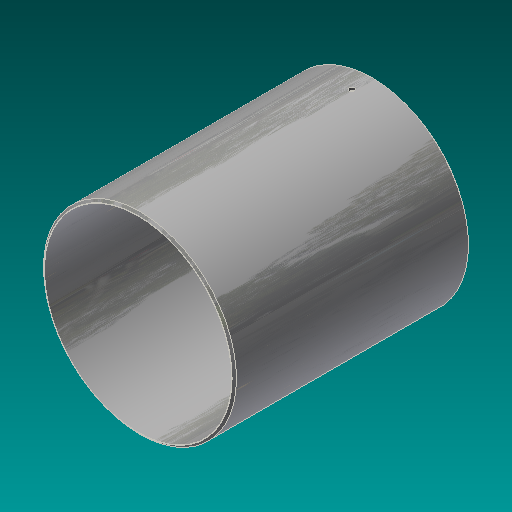
# Autodesk Inventor part: A1-19027-200-01 34in pipe
Saved by Autodesk Inventor 2017.3 (Build 213257000, 257)
## iProperties
Created: 2019-06-26
Part Number: A1-19027-200-01 34in pipe
Material: Steel, Mild
Document SubType Name: Modeling
Designer: Graeme_Van_Dongen
Density: 7.85 g/cm^3
Appearance: Steel
Mass: 279198 g
Surface Area: 56801.7 cm^2
Volume: 35566.7 cm^3
Description: 34" XS x 41 9/16" PIPE, API 5L X65M
Author: Graeme_Van_Dongen
Autodesk Inventor part; units mm, degrees
ref_plane "YZ Plane" through (0, 0, 0) normal (1, 0, 0) x (0, 1, 0)
ref_plane "XY Plane" through (0, 0, 0) normal (0, 0, 1) x (1, 0, 0)
sketch "Sketch1" plane through (0, 0, 0) normal (0, 0, 1) x (1, 0, 0)
  circle A0 centre (0, 0) radius 431.8
  circle A1 centre (0, 0) radius 419.1
  dimension "d0" = 863.6
  dimension "d1" = 838.2
  constraints: 2 centre point, 2 coincident
  measures "d0" diameter of A0
  measures "d1" diameter of A1
extrude "Extrusion1" add sketch "Sketch1" along normal blind 1055.4625
chamfer "Chamfer1" distance 11.1125 angle 37.5 1 edges at (-431.8, 0, 0) measured on face at (-431.3, 0, 0)
chamfer "Chamfer2" distance 11.1125 angle 37.5 1 edges at (-431.8, 0, 1055.4625) measured on face at (-431.3, 0, 1055.4625)
ref_plane "Work Plane1" through (0, 431.8, 0) normal (0, 1, 0) x (-1, 0, 0)
sketch "Sketch2" plane through (0, 431.8, 0) normal (0, 1, 0) x (-1, 0, 0)
  point P0 (0, 0)
  point P1 (0, 99.2188)
  dimension "d10" = 99.2188
  constraints: 1 vertical alignment
  measures "d10" distance of point (0, 0) point (0, 99.219)
hole "Hole1" at (0, 431.8, 99.2188) direction (0, -1, 0) diameter 22.6314 depth 23.114 tip angle 118 taper from width 23.6614 to width 22.7838 over 14.0462 thread size "3/4" designation "3/4 - 14 NPT" standard "NPT"
pattern_circular "Circular Pattern1" count 2 over 360 about axis through (0, 0, -10) along (0, 0, 1) of "Hole1"
equation "\"d7\" = d4"
equation "\"d9\" = d6"
equation "\"d4\" = 11.1125"
equation "\"d6\" = 37.5deg"
body "Solid1"
